Autodesk Fusion 360 part; units mm, degrees
(part 3 of 8)
  spline S623 degree 3 poles (3.0732, -97.2295) (3.0688, -97.132) (3.0596, -97.098) (3.0422, -97.1202) knots 0 0 0 0 1 1 1 1
  spline S624 degree 3 poles (3.0422, -97.1202) (3.0378, -97.1258) (3.0439, -97.1753) (3.0534, -97.2319) knots 0 0 0 0 1 1 1 1
  spline S625 degree 3 poles (10.0535, -88.2722) (10.072, -88.3001) (10.1317, -88.3154) (10.1877, -88.301) knots 0 0 0 0 1 1 1 1
  spline S626 degree 3 poles (10.1877, -88.301) (10.2366, -88.2899) (10.2509, -88.2832) (10.2156, -88.2825) knots 0 0 0 0 1 1 1 1
  spline S627 degree 3 poles (10.2156, -88.2825) (10.1259, -88.2885) (10.0814, -88.2537) (10.1572, -88.2368) knots 0 0 0 0 1 1 1 1
  spline S628 degree 3 poles (10.1572, -88.2368) (10.1913, -88.2276) (10.217, -88.2119) (10.2152, -88.1971) knots 0 0 0 0 1 1 1 1
  spline S629 degree 3 poles (10.2152, -88.1971) (10.2133, -88.1822) (10.2474, -88.173) (10.2898, -88.1703) knots 0 0 0 0 1 1 1 1
  spline S630 degree 3 poles (10.2898, -88.1703) (10.3625, -88.1689) (10.3631, -88.1739) (10.2944, -88.1873) knots 0 0 0 0 1 1 1 1
  spline S631 degree 3 poles (10.2944, -88.1873) (10.1851, -88.2183) (10.2327, -88.2376) (10.4091, -88.2411) knots 0 0 0 0 1 1 1 1
  spline S632 degree 3 poles (10.4091, -88.2411) (10.4895, -88.2413) (10.5632, -88.2272) (10.5635, -88.2096) knots 0 0 0 0 1 1 1 1
  spline S633 degree 3 poles (10.5635, -88.2096) (10.566, -88.1892) (10.5846, -88.1768) (10.61, -88.1787) knots 0 0 0 0 1 1 1 1
  spline S634 degree 3 poles (10.61, -88.1787) (10.6354, -88.1807) (10.6561, -88.1655) (10.6559, -88.1429) knots 0 0 0 0 1 1 1 1
  spline S635 degree 3 poles (10.6559, -88.1429) (10.6593, -88.1099) (10.2729, -88.0945) (10.2138, -88.1243) knots 0 0 0 0 1 1 1 1
  spline S636 degree 3 poles (10.2138, -88.1243) (10.1974, -88.1339) (10.1686, -88.1249) (10.1464, -88.1075) knots 0 0 0 0 1 1 1 1
  spline S637 degree 3 poles (10.1464, -88.1075) (10.0908, -88.0641) (10.0032, -88.2105) (10.0535, -88.2722) knots 0 0 0 0 1 1 1 1
  spline S638 degree 3 poles (10.2393, -88.0458) (10.2449, -88.0502) (10.2845, -88.0453) (10.3257, -88.0327) knots 0 0 0 0 1 1 1 1
  spline S639 degree 3 poles (10.3257, -88.0327) (10.3944, -88.0192) (10.3938, -88.0143) (10.3211, -88.0157) knots 0 0 0 0 1 1 1 1
  spline S640 degree 3 poles (10.3211, -88.0157) (10.2483, -88.0171) (10.2171, -88.0284) (10.2393, -88.0458) knots 0 0 0 0 1 1 1 1
  line L60 (3.056, -97.4578) -> (3.0787, -97.5606)
  line L61 (3.0787, -97.5606) -> (3.0758, -97.4554)
  spline S641 degree 3 poles (3.0758, -97.4554) (3.0713, -97.3981) (3.0652, -97.3486) (3.0596, -97.3442) knots 0 0 0 0 1 1 1 1
  spline S642 degree 3 poles (3.0596, -97.3442) (3.0374, -97.3269) (3.0367, -97.3621) (3.056, -97.4578) knots 0 0 0 0 1 1 1 1
  spline S643 degree 3 poles (10.0643, -88.4016) (10.081, -88.4146) (10.129, -88.4162) (10.1702, -88.4036) knots 0 0 0 0 1 1 1 1
  spline S644 degree 3 poles (10.1702, -88.4036) (10.241, -88.3874) (10.241, -88.3874) (10.1578, -88.3851) knots 0 0 0 0 1 1 1 1
  spline S645 degree 3 poles (10.1578, -88.3851) (10.1099, -88.3834) (10.0619, -88.3818) (10.0542, -88.3802) knots 0 0 0 0 1 1 1 1
  spline S646 degree 3 poles (10.0542, -88.3802) (10.0443, -88.3814) (10.0477, -88.3885) (10.0643, -88.4016) knots 0 0 0 0 1 1 1 1
  spline S647 degree 3 poles (3.0556, -97.6589) (3.0718, -97.7298) (3.0768, -97.7292) (3.0754, -97.6565) knots 0 0 0 0 1 1 1 1
  spline S648 degree 3 poles (3.0754, -97.6565) (3.0755, -97.6162) (3.0706, -97.5766) (3.065, -97.5723) knots 0 0 0 0 1 1 1 1
  spline S649 degree 3 poles (3.065, -97.5723) (3.0428, -97.5549) (3.0393, -97.588) (3.0556, -97.6589) knots 0 0 0 0 1 1 1 1
  spline S650 degree 3 poles (10.9708, -87.4533) (10.9764, -87.4577) (11.016, -87.4528) (11.0572, -87.4402) knots 0 0 0 0 1 1 1 1
  spline S651 degree 3 poles (11.0572, -87.4402) (11.1259, -87.4268) (11.1253, -87.4218) (11.0526, -87.4232) knots 0 0 0 0 1 1 1 1
  spline S652 degree 3 poles (11.0526, -87.4232) (10.9798, -87.4246) (10.9486, -87.436) (10.9708, -87.4533) knots 0 0 0 0 1 1 1 1
  spline S653 degree 3 poles (10.2069, -88.5801) (10.3192, -88.5738) (10.3329, -88.5621) (10.2648, -88.5403) knots 0 0 0 0 1 1 1 1
  spline S654 degree 3 poles (10.2648, -88.5403) (10.2361, -88.5313) (10.1894, -88.5395) (10.1587, -88.5559) knots 0 0 0 0 1 1 1 1
  spline S655 degree 3 poles (10.1587, -88.5559) (10.1165, -88.5811) (10.1249, -88.5876) (10.2069, -88.5801) knots 0 0 0 0 1 1 1 1
  spline S656 degree 3 poles (3.0521, -97.8353) (3.0683, -97.9061) (3.0733, -97.9055) (3.0719, -97.8328) knots 0 0 0 0 1 1 1 1
  spline S657 degree 3 poles (3.0719, -97.8328) (3.072, -97.7926) (3.0671, -97.753) (3.0616, -97.7486) knots 0 0 0 0 1 1 1 1
  spline S658 degree 3 poles (3.0616, -97.7486) (3.0393, -97.7313) (3.0358, -97.7644) (3.0521, -97.8353) knots 0 0 0 0 1 1 1 1
  spline S659 degree 3 poles (11.3124, -87.4516) (11.4105, -87.4521) (11.4974, -87.444) (11.504, -87.4356) knots 0 0 0 0 1 1 1 1
  spline S660 degree 3 poles (11.504, -87.4356) (11.5083, -87.4301) (11.4322, -87.4243) (11.3341, -87.4238) knots 0 0 0 0 1 1 1 1
  spline S661 degree 3 poles (11.3341, -87.4238) (11.236, -87.4233) (11.1491, -87.4315) (11.1426, -87.4398) knots 0 0 0 0 1 1 1 1
  spline S662 degree 3 poles (11.1426, -87.4398) (11.1382, -87.4454) (11.2143, -87.4511) (11.3124, -87.4516) knots 0 0 0 0 1 1 1 1
  spline S663 degree 3 poles (10.5969, -88.2356) (10.6108, -88.2465) (10.6665, -88.2497) (10.7182, -88.2409) knots 0 0 0 0 1 1 1 1
  spline S664 degree 3 poles (10.7182, -88.2409) (10.7699, -88.232) (10.8005, -88.2157) (10.7894, -88.207) knots 0 0 0 0 1 1 1 1
  spline S665 degree 3 poles (10.7894, -88.207) (10.7783, -88.1983) (10.8089, -88.182) (10.8606, -88.1731) knots 0 0 0 0 1 1 1 1
  spline S666 degree 3 poles (10.8606, -88.1731) (10.9123, -88.1642) (10.9652, -88.1653) (10.9819, -88.1783) knots 0 0 0 0 1 1 1 1
  spline S667 degree 3 poles (10.9819, -88.1783) (10.9958, -88.1892) (10.9596, -88.2012) (10.8974, -88.2063) knots 0 0 0 0 1 1 1 1
  spline S668 degree 3 poles (10.8974, -88.2063) (10.7575, -88.2134) (10.8531, -88.2343) (11.0471, -88.2382) knots 0 0 0 0 1 1 1 1
  spline S669 degree 3 poles (11.0471, -88.2382) (11.1275, -88.2383) (11.1891, -88.2283) (11.1873, -88.2134) knots 0 0 0 0 1 1 1 1
  spline S670 degree 3 poles (11.1873, -88.2134) (11.1855, -88.1986) (11.2232, -88.1788) (11.2728, -88.1728) knots 0 0 0 0 1 1 1 1
  spline S671 degree 3 poles (11.2728, -88.1728) (11.3514, -88.1581) (11.3536, -88.1553) (11.3119, -88.1227) knots 0 0 0 0 1 1 1 1
  spline S672 degree 3 poles (11.3119, -88.1227) (11.2841, -88.101) (11.2581, -88.0941) (11.2494, -88.1053) knots 0 0 0 0 1 1 1 1
  spline S673 degree 3 poles (11.2494, -88.1053) (11.2385, -88.1192) (11.1135, -88.1245) (10.9675, -88.1223) knots 0 0 0 0 1 1 1 1
  spline S674 degree 3 poles (10.9675, -88.1223) (10.8236, -88.1173) (10.6964, -88.1254) (10.6856, -88.1393) knots 0 0 0 0 1 1 1 1
  spline S675 degree 3 poles (10.6856, -88.1393) (10.6769, -88.1504) (10.6914, -88.1662) (10.7168, -88.1681) knots 0 0 0 0 1 1 1 1
  spline S676 degree 3 poles (10.7168, -88.1681) (10.7449, -88.1722) (10.7235, -88.1824) (10.6697, -88.194) knots 0 0 0 0 1 1 1 1
  spline S677 degree 3 poles (10.6697, -88.194) (10.613, -88.2035) (10.5802, -88.2226) (10.5969, -88.2356) knots 0 0 0 0 1 1 1 1
  line L62 (3.0493, -98.1196) -> (3.0625, -98.309)
  line L63 (3.0625, -98.309) -> (3.0669, -98.1199)
  spline S678 degree 3 poles (3.0669, -98.1199) (3.0701, -97.9612) (3.0622, -97.8968) (3.0426, -97.9219) knots 0 0 0 0 1 1 1 1
  spline S679 degree 3 poles (3.0426, -97.9219) (3.0383, -97.9274) (3.0415, -98.015) (3.0493, -98.1196) knots 0 0 0 0 1 1 1 1
  spline S680 degree 3 poles (10.3783, -88.5842) (10.4114, -88.5877) (10.4321, -88.6128) (10.4286, -88.6459) knots 0 0 0 0 1 1 1 1
  spline S681 degree 3 poles (10.4286, -88.6459) (10.4251, -88.679) (10.4341, -88.6904) (10.4449, -88.6765) knots 0 0 0 0 1 1 1 1
  spline S682 degree 3 poles (10.4449, -88.6765) (10.458, -88.6598) (10.4686, -88.6234) (10.4699, -88.593) knots 0 0 0 0 1 1 1 1
  spline S683 degree 3 poles (10.4699, -88.593) (10.4749, -88.5522) (10.4588, -88.5441) (10.4, -88.5564) knots 0 0 0 0 1 1 1 1
  spline S684 degree 3 poles (10.4, -88.5564) (10.339, -88.5714) (10.3347, -88.577) (10.3783, -88.5842) knots 0 0 0 0 1 1 1 1
  spline S685 degree 3 poles (7.4661, -92.4377) (7.4741, -92.4618) (7.4886, -92.4776) (7.5035, -92.4758) knots 0 0 0 0 1 1 1 1
  spline S686 degree 3 poles (7.5035, -92.4758) (7.5161, -92.4768) (7.5131, -92.452) (7.4946, -92.4241) knots 0 0 0 0 1 1 1 1
  spline S687 degree 3 poles (7.4946, -92.4241) (7.4625, -92.3677) (7.4412, -92.3779) (7.4661, -92.4377) knots 0 0 0 0 1 1 1 1
  spline S688 degree 3 poles (10.8674, -88.0441) (10.873, -88.0484) (10.9126, -88.0436) (10.9538, -88.031) knots 0 0 0 0 1 1 1 1
  spline S689 degree 3 poles (10.9538, -88.031) (11.0225, -88.0175) (11.0219, -88.0126) (10.9492, -88.0139) knots 0 0 0 0 1 1 1 1
  spline S690 degree 3 poles (10.9492, -88.0139) (10.8765, -88.0153) (10.8452, -88.0267) (10.8674, -88.0441) knots 0 0 0 0 1 1 1 1
  spline S691 degree 3 poles (10.546, -88.5988) (10.5626, -88.6118) (10.5908, -88.6159) (10.6122, -88.6057) knots 0 0 0 0 1 1 1 1
  spline S692 degree 3 poles (10.6122, -88.6057) (10.6335, -88.5956) (10.6246, -88.5841) (10.5958, -88.5751) knots 0 0 0 0 1 1 1 1
  spline S693 degree 3 poles (10.5958, -88.5751) (10.5306, -88.5554) (10.507, -88.5684) (10.546, -88.5988) knots 0 0 0 0 1 1 1 1
  spline S694 degree 3 poles (10.1038, -89.1934) (10.1093, -89.1978) (10.1489, -89.1929) (10.1901, -89.1803) knots 0 0 0 0 1 1 1 1
  spline S695 degree 3 poles (10.1901, -89.1803) (10.2588, -89.1668) (10.2582, -89.1619) (10.1855, -89.1633) knots 0 0 0 0 1 1 1 1
  spline S696 degree 3 poles (10.1855, -89.1633) (10.1128, -89.1647) (10.0815, -89.176) (10.1038, -89.1934) knots 0 0 0 0 1 1 1 1
  spline S697 degree 3 poles (3.0484, -98.5218) (3.0583, -98.6639) (3.0651, -98.6781) (3.0733, -98.5816) knots 0 0 0 0 1 1 1 1
  spline S698 degree 3 poles (3.0733, -98.5816) (3.0813, -98.4625) (3.0607, -98.2941) (3.0439, -98.3213) knots 0 0 0 0 1 1 1 1
  spline S699 degree 3 poles (3.0439, -98.3213) (3.0423, -98.329) (3.0434, -98.4194) (3.0484, -98.5218) knots 0 0 0 0 1 1 1 1
  spline S700 degree 3 poles (11.6264, -87.4508) (11.6787, -87.4468) (11.7255, -87.4386) (11.732, -87.4303) knots 0 0 0 0 1 1 1 1
  spline S701 degree 3 poles (11.732, -87.4303) (11.7385, -87.4219) (11.7005, -87.419) (11.6482, -87.423) knots 0 0 0 0 1 1 1 1
  spline S702 degree 3 poles (11.6482, -87.423) (11.5959, -87.4269) (11.5491, -87.4351) (11.5426, -87.4435) knots 0 0 0 0 1 1 1 1
  spline S703 degree 3 poles (11.5426, -87.4435) (11.5361, -87.4518) (11.5741, -87.4547) (11.6264, -87.4508) knots 0 0 0 0 1 1 1 1
  spline S704 degree 3 poles (11.9405, -87.4499) (12.0386, -87.4504) (12.1255, -87.4423) (12.1321, -87.4339) knots 0 0 0 0 1 1 1 1
  spline S705 degree 3 poles (12.1321, -87.4339) (12.1364, -87.4284) (12.0603, -87.4226) (11.9622, -87.4221) knots 0 0 0 0 1 1 1 1
  spline S706 degree 3 poles (11.9622, -87.4221) (11.8641, -87.4216) (11.7772, -87.4297) (11.7707, -87.4381) knots 0 0 0 0 1 1 1 1
  spline S707 degree 3 poles (11.7707, -87.4381) (11.7663, -87.4436) (11.8424, -87.4494) (11.9405, -87.4499) knots 0 0 0 0 1 1 1 1
  spline S708 degree 3 poles (11.225, -88.2339) (11.2611, -88.2622) (11.4261, -88.2344) (11.4191, -88.1975) knots 0 0 0 0 1 1 1 1
  spline S709 degree 3 poles (11.4191, -88.1975) (11.4164, -88.1551) (11.649, -88.1668) (11.6771, -88.2111) knots 0 0 0 0 1 1 1 1
  spline S710 degree 3 poles (11.6771, -88.2111) (11.69, -88.2346) (11.7342, -88.2468) (11.7732, -88.237) knots 0 0 0 0 1 1 1 1
  spline S711 degree 3 poles (11.7732, -88.237) (11.8101, -88.2299) (11.8308, -88.2148) (11.8197, -88.2061) knots 0 0 0 0 1 1 1 1
  spline S712 degree 3 poles (11.8197, -88.2061) (11.8058, -88.1953) (11.8393, -88.1811) (11.891, -88.1723) knots 0 0 0 0 1 1 1 1
  spline S713 degree 3 poles (11.891, -88.1723) (11.9943, -88.1545) (11.9657, -88.1053) (11.8589, -88.1159) knots 0 0 0 0 1 1 1 1
  spline S714 degree 3 poles (11.8589, -88.1159) (11.8242, -88.1201) (11.7262, -88.1196) (11.6451, -88.1145) knots 0 0 0 0 1 1 1 1
  spline S715 degree 3 poles (11.6451, -88.1145) (11.4428, -88.1041) (11.3586, -88.1145) (11.3656, -88.1513) knots 0 0 0 0 1 1 1 1
  spline S716 degree 3 poles (11.3656, -88.1513) (11.3653, -88.1689) (11.3303, -88.1908) (11.2808, -88.1969) knots 0 0 0 0 1 1 1 1
  spline S717 degree 3 poles (11.2808, -88.1969) (11.234, -88.2052) (11.2083, -88.2209) (11.225, -88.2339) knots 0 0 0 0 1 1 1 1
  spline S718 degree 3 poles (3.0529, -98.8656) (3.0692, -98.9365) (3.0741, -98.9359) (3.0727, -98.8631) knots 0 0 0 0 1 1 1 1
  spline S719 degree 3 poles (3.0727, -98.8631) (3.0728, -98.8229) (3.068, -98.7833) (3.0624, -98.779) knots 0 0 0 0 1 1 1 1
  spline S720 degree 3 poles (3.0624, -98.779) (3.0402, -98.7616) (3.0367, -98.7947) (3.0529, -98.8656) knots 0 0 0 0 1 1 1 1
  spline S721 degree 3 poles (11.446, -88.0484) (11.4516, -88.0528) (11.4912, -88.0479) (11.5324, -88.0353) knots 0 0 0 0 1 1 1 1
  spline S722 degree 3 poles (11.5324, -88.0353) (11.6011, -88.0219) (11.6005, -88.0169) (11.5277, -88.0183) knots 0 0 0 0 1 1 1 1
  spline S723 degree 3 poles (11.5277, -88.0183) (11.455, -88.0197) (11.4238, -88.0311) (11.446, -88.0484) knots 0 0 0 0 1 1 1 1
  spline S724 degree 3 poles (11.2364, -88.5115) (11.2503, -88.5223) (11.2933, -88.5246) (11.3302, -88.5176) knots 0 0 0 0 1 1 1 1
  spline S725 degree 3 poles (11.3302, -88.5176) (11.367, -88.5105) (11.385, -88.4932) (11.3683, -88.4802) knots 0 0 0 0 1 1 1 1
  spline S726 degree 3 poles (11.3683, -88.4802) (11.3544, -88.4694) (11.3114, -88.4671) (11.2746, -88.4741) knots 0 0 0 0 1 1 1 1
  spline S727 degree 3 poles (11.2746, -88.4741) (11.2378, -88.4812) (11.2198, -88.4985) (11.2364, -88.5115) knots 0 0 0 0 1 1 1 1
  spline S728 degree 3 poles (11.4536, -88.2335) (11.4675, -88.2443) (11.5226, -88.2426) (11.5771, -88.2359) knots 0 0 0 0 1 1 1 1
  spline S729 degree 3 poles (11.5771, -88.2359) (11.6777, -88.216) (11.6777, -88.216) (11.5905, -88.2016) knots 0 0 0 0 1 1 1 1
  spline S730 degree 3 poles (11.5905, -88.2016) (11.4977, -88.1828) (11.4147, -88.2031) (11.4536, -88.2335) knots 0 0 0 0 1 1 1 1
  spline S731 degree 3 poles (3.0555, -99.0915) (3.0718, -99.1623) (3.0767, -99.1617) (3.0753, -99.089) knots 0 0 0 0 1 1 1 1
  spline S732 degree 3 poles (3.0753, -99.089) (3.0754, -99.0488) (3.0706, -99.0092) (3.065, -99.0048) knots 0 0 0 0 1 1 1 1
  spline S733 degree 3 poles (3.065, -99.0048) (3.0428, -98.9875) (3.0393, -99.0206) (3.0555, -99.0915) knots 0 0 0 0 1 1 1 1
  spline S734 degree 3 poles (11.0982, -88.7572) (11.1205, -88.7745) (11.1681, -88.7938) (11.2012, -88.7973) knots 0 0 0 0 1 1 1 1
  spline S735 degree 3 poles (11.2012, -88.7973) (11.2773, -88.803) (11.2328, -88.7683) (11.1317, -88.743) knots 0 0 0 0 1 1 1 1
  spline S736 degree 3 poles (11.1317, -88.743) (11.0825, -88.7314) (11.0704, -88.7354) (11.0982, -88.7572) knots 0 0 0 0 1 1 1 1
  spline S737 degree 3 poles (11.6719, -88.0458) (11.6774, -88.0502) (11.717, -88.0453) (11.7582, -88.0327) knots 0 0 0 0 1 1 1 1
  spline S738 degree 3 poles (11.7582, -88.0327) (11.8269, -88.0193) (11.8263, -88.0143) (11.7536, -88.0157) knots 0 0 0 0 1 1 1 1
  spline S739 degree 3 poles (11.7536, -88.0157) (11.6809, -88.0171) (11.6496, -88.0285) (11.6719, -88.0458) knots 0 0 0 0 1 1 1 1
  spline S740 degree 3 poles (12.0628, -87.5455) (12.0684, -87.5498) (12.108, -87.5449) (12.1492, -87.5323) knots 0 0 0 0 1 1 1 1
  spline S741 degree 3 poles (12.1492, -87.5323) (12.2179, -87.5189) (12.2173, -87.5139) (12.1446, -87.5153) knots 0 0 0 0 1 1 1 1
  spline S742 degree 3 poles (12.1446, -87.5153) (12.0719, -87.5167) (12.0406, -87.5281) (12.0628, -87.5455) knots 0 0 0 0 1 1 1 1
  spline S743 degree 3 poles (12.503, -87.4462) (12.697, -87.45) (12.9306, -87.449) (13.0203, -87.443) knots 0 0 0 0 1 1 1 1
  spline S744 degree 3 poles (13.0203, -87.443) (13.1101, -87.437) (13.0263, -87.4297) (12.8323, -87.4259) knots 0 0 0 0 1 1 1 1
  spline S745 degree 3 poles (12.8323, -87.4259) (12.6383, -87.422) (12.4047, -87.4231) (12.3149, -87.4291) knots 0 0 0 0 1 1 1 1
  spline S746 degree 3 poles (12.3149, -87.4291) (12.223, -87.4378) (12.309, -87.4423) (12.503, -87.4462) knots 0 0 0 0 1 1 1 1
  spline S747 degree 3 poles (3.052, -99.2678) (3.0683, -99.3387) (3.0732, -99.3381) (3.0719, -99.2654) knots 0 0 0 0 1 1 1 1
  spline S748 degree 3 poles (3.0719, -99.2654) (3.0719, -99.2252) (3.0671, -99.1855) (3.0615, -99.1812) knots 0 0 0 0 1 1 1 1
  spline S749 degree 3 poles (3.0615, -99.1812) (3.0393, -99.1638) (3.0358, -99.1969) (3.052, -99.2678) knots 0 0 0 0 1 1 1 1
  line L64 (3.0516, -99.4689) -> (3.0743, -99.5717)
  line L65 (3.0743, -99.5717) -> (3.0714, -99.4665)
  spline S750 degree 3 poles (3.0714, -99.4665) (3.067, -99.369) (3.0578, -99.335) (3.0404, -99.3572) knots 0 0 0 0 1 1 1 1
  spline S751 degree 3 poles (3.0404, -99.3572) (3.0361, -99.3628) (3.0421, -99.4123) (3.0516, -99.4689) knots 0 0 0 0 1 1 1 1
  spline S752 degree 3 poles (11.8977, -88.0432) (11.9033, -88.0476) (11.9429, -88.0427) (11.9841, -88.0301) knots 0 0 0 0 1 1 1 1
  spline S753 degree 3 poles (11.9841, -88.0301) (12.0528, -88.0167) (12.0522, -88.0117) (11.9795, -88.0131) knots 0 0 0 0 1 1 1 1
  spline S754 degree 3 poles (11.9795, -88.0131) (11.9068, -88.0145) (11.8755, -88.0259) (11.8977, -88.0432) knots 0 0 0 0 1 1 1 1
  spline S755 degree 3 poles (11.8531, -88.2322) (11.867, -88.2431) (11.9227, -88.2463) (11.9744, -88.2374) knots 0 0 0 0 1 1 1 1
  spline S756 degree 3 poles (11.9744, -88.2374) (12.0261, -88.2286) (12.0567, -88.2122) (12.0456, -88.2035) knots 0 0 0 0 1 1 1 1
  spline S757 degree 3 poles (12.0456, -88.2035) (12.0345, -88.1948) (12.0651, -88.1785) (12.1168, -88.1697) knots 0 0 0 0 1 1 1 1
  spline S758 degree 3 poles (12.1168, -88.1697) (12.2252, -88.1513) (12.1977, -88.112) (12.0715, -88.1074) knots 0 0 0 0 1 1 1 1
  spline S759 degree 3 poles (12.0715, -88.1074) (12.0263, -88.1079) (11.9879, -88.1227) (11.9931, -88.1446) knots 0 0 0 0 1 1 1 1
  spline S760 degree 3 poles (11.9931, -88.1446) (11.9956, -88.1644) (11.9584, -88.1891) (11.9089, -88.1952) knots 0 0 0 0 1 1 1 1
  spline S761 degree 3 poles (11.9089, -88.1952) (11.8621, -88.2034) (11.8364, -88.2192) (11.8531, -88.2322) knots 0 0 0 0 1 1 1 1
  line L66 (3.0542, -99.6948) -> (3.0769, -99.7976)
  line L67 (3.0769, -99.7976) -> (3.074, -99.6924)
  spline S762 degree 3 poles (3.074, -99.6924) (3.0696, -99.5949) (3.0604, -99.5608) (3.043, -99.5831) knots 0 0 0 0 1 1 1 1
  spline S763 degree 3 poles (3.043, -99.5831) (3.0387, -99.5886) (3.0447, -99.6382) (3.0542, -99.6948) knots 0 0 0 0 1 1 1 1
  spline S764 degree 3 poles (12.0741, -88.0467) (12.0797, -88.0511) (12.1193, -88.0462) (12.1605, -88.0336) knots 0 0 0 0 1 1 1 1
  spline S765 degree 3 poles (12.1605, -88.0336) (12.2292, -88.0201) (12.2286, -88.0152) (12.1558, -88.0166) knots 0 0 0 0 1 1 1 1
  spline S766 degree 3 poles (12.1558, -88.0166) (12.0831, -88.018) (12.0519, -88.0293) (12.0741, -88.0467) knots 0 0 0 0 1 1 1 1
  spline S767 degree 3 poles (12.0706, -88.2231) (12.1095, -88.2535) (12.4422, -88.2403) (12.4478, -88.2044) knots 0 0 0 0 1 1 1 1
  spline S768 degree 3 poles (12.4478, -88.2044) (12.4482, -88.1868) (12.4866, -88.172) (12.5296, -88.1743) knots 0 0 0 0 1 1 1 1
  spline S769 degree 3 poles (12.5296, -88.1743) (12.5995, -88.1707) (12.6001, -88.1757) (12.5314, -88.1891) knots 0 0 0 0 1 1 1 1
  spline S770 degree 3 poles (12.5314, -88.1891) (12.4902, -88.2017) (12.4673, -88.2196) (12.484, -88.2326) knots 0 0 0 0 1 1 1 1
  spline S771 degree 3 poles (12.484, -88.2326) (12.5173, -88.2587) (12.6328, -88.237) (12.6285, -88.2023) knots 0 0 0 0 1 1 1 1
  spline S772 degree 3 poles (12.6285, -88.2023) (12.6267, -88.1875) (12.6608, -88.1783) (12.7032, -88.1756) knots 0 0 0 0 1 1 1 1
  spline S773 degree 3 poles (12.7032, -88.1756) (12.7759, -88.1742) (12.7765, -88.1791) (12.7078, -88.1926) knots 0 0 0 0 1 1 1 1
  spline S774 degree 3 poles (12.7078, -88.1926) (12.6666, -88.2052) (12.6436, -88.2231) (12.6603, -88.2361) knots 0 0 0 0 1 1 1 1
  spline S775 degree 3 poles (12.6603, -88.2361) (12.6937, -88.2622) (12.8091, -88.2405) (12.8049, -88.2058) knots 0 0 0 0 1 1 1 1
  spline S776 degree 3 poles (12.8049, -88.2058) (12.8031, -88.191) (12.8371, -88.1817) (12.8795, -88.1791) knots 0 0 0 0 1 1 1 1
  spline S777 degree 3 poles (12.8795, -88.1791) (12.9522, -88.1777) (12.9528, -88.1826) (12.8841, -88.1961) knots 0 0 0 0 1 1 1 1
  spline S778 degree 3 poles (12.8841, -88.1961) (12.8429, -88.2087) (12.82, -88.2266) (12.8339, -88.2374) knots 0 0 0 0 1 1 1 1
  spline S779 degree 3 poles (12.8339, -88.2374) (12.8756, -88.27) (13.0344, -88.2329) (13.0295, -88.1933) knots 0 0 0 0 1 1 1 1
  spline S780 degree 3 poles (13.0295, -88.1933) (13.0271, -88.1735) (13.041, -88.1844) (13.0629, -88.2194) knots 0 0 0 0 1 1 1 1
  spline S781 degree 3 poles (13.0629, -88.2194) (13.0977, -88.2779) (13.0956, -88.2807) (13.0068, -88.274) knots 0 0 0 0 1 1 1 1
  spline S782 degree 3 poles (13.0068, -88.274) (12.956, -88.2702) (12.9043, -88.279) (12.8935, -88.2929) knots 0 0 0 0 1 1 1 1
  spline S783 degree 3 poles (12.8935, -88.2929) (12.8826, -88.3068) (13.0194, -88.3152) (13.1923, -88.3115) knots 0 0 0 0 1 1 1 1
  spline S784 degree 3 poles (13.1923, -88.3115) (13.3681, -88.3101) (13.5095, -88.2952) (13.5077, -88.2804) knots 0 0 0 0 1 1 1 1
  spline S785 degree 3 poles (13.5077, -88.2804) (13.5059, -88.2655) (13.5437, -88.2458) (13.5932, -88.2397) knots 0 0 0 0 1 1 1 1
  spline S786 degree 3 poles (13.5932, -88.2397) (13.6399, -88.2315) (13.6684, -88.2179) (13.6545, -88.207) knots 0 0 0 0 1 1 1 1
  spline S787 degree 3 poles (13.6545, -88.207) (13.6434, -88.1984) (13.6642, -88.1832) (13.701, -88.1762) knots 0 0 0 0 1 1 1 1
  spline S788 degree 3 poles (13.701, -88.1762) (13.7549, -88.1646) (13.7614, -88.1562) (13.7308, -88.1323) knots 0 0 0 0 1 1 1 1
  spline S789 degree 3 poles (13.7308, -88.1323) (13.673, -88.0917) (13.4341, -88.111) (13.4099, -88.1592) knots 0 0 0 0 1 1 1 1
  spline S790 degree 3 poles (13.4099, -88.1592) (13.4024, -88.1802) (13.3705, -88.1866) (13.3461, -88.172) knots 0 0 0 0 1 1 1 1
  spline S791 degree 3 poles (13.3461, -88.172) (13.3239, -88.1546) (13.2834, -88.132) (13.2611, -88.1146) knots 0 0 0 0 1 1 1 1
  spline S792 degree 3 poles (13.2611, -88.1146) (13.2395, -88.1022) (13.2132, -88.1129) (13.202, -88.1445) knots 0 0 0 0 1 1 1 1
  spline S793 degree 3 poles (13.202, -88.1445) (13.1957, -88.1754) (13.1678, -88.1939) (13.1425, -88.192) knots 0 0 0 0 1 1 1 1
  spline S794 degree 3 poles (13.1425, -88.192) (13.1143, -88.1879) (13.1137, -88.183) (13.14, -88.1722) knots 0 0 0 0 1 1 1 1
  spline S795 degree 3 poles (13.14, -88.1722) (13.1664, -88.1614) (13.1772, -88.1475) (13.1633, -88.1367) knots 0 0 0 0 1 1 1 1
  spline S796 degree 3 poles (13.1633, -88.1367) (13.125, -88.1112) (12.9363, -88.0891) (12.9647, -88.1158) knots 0 0 0 0 1 1 1 1
  spline S797 degree 3 poles (12.9647, -88.1158) (12.9786, -88.1267) (12.9341, -88.1321) (12.8623, -88.1208) knots 0 0 0 0 1 1 1 1
  spline S798 degree 3 poles (12.8623, -88.1208) (12.7299, -88.1069) (12.617, -88.1082) (12.4149, -88.1205) knots 0 0 0 0 1 1 1 1
  spline S799 degree 3 poles (12.4149, -88.1205) (12.3499, -88.1234) (12.2794, -88.122) (12.2584, -88.1146) knots 0 0 0 0 1 1 1 1
  spline S800 degree 3 poles (12.2584, -88.1146) (12.2346, -88.1049) (12.216, -88.1173) (12.2184, -88.1371) knots 0 0 0 0 1 1 1 1
  spline S801 degree 3 poles (12.2184, -88.1371) (12.2208, -88.1569) (12.2458, -88.1764) (12.2789, -88.1799) knots 0 0 0 0 1 1 1 1
  spline S802 degree 3 poles (12.2789, -88.1799) (12.3093, -88.1812) (12.2696, -88.1861) (12.1898, -88.1909) knots 0 0 0 0 1 1 1 1
  spline S803 degree 3 poles (12.1898, -88.1909) (12.1128, -88.1978) (12.0567, -88.2122) (12.0706, -88.2231) knots 0 0 0 0 1 1 1 1
  spline S804 degree 3 poles (13.2554, -88.1907) (13.253, -88.1709) (13.2641, -88.1796) (13.2798, -88.2053) knots 0 0 0 0 1 1 1 1
  spline S805 degree 3 poles (13.2798, -88.2053) (13.2983, -88.2332) (13.3432, -88.2503) (13.3822, -88.2405) knots 0 0 0 0 1 1 1 1
  spline S806 degree 3 poles (13.3822, -88.2405) (13.419, -88.2334) (13.4648, -88.2379) (13.4815, -88.2509) knots 0 0 0 0 1 1 1 1
  spline S807 degree 3 poles (13.4815, -88.2509) (13.4981, -88.2639) (13.4272, -88.2802) (13.3248, -88.2852) knots 0 0 0 0 1 1 1 1
  spline S808 degree 3 poles (13.3248, -88.2852) (13.1271, -88.2919) (13.0309, -88.266) (13.1711, -88.2413) knots 0 0 0 0 1 1 1 1
  spline S809 degree 3 poles (13.1711, -88.2413) (13.2207, -88.2352) (13.2578, -88.2105) (13.2554, -88.1907) knots 0 0 0 0 1 1 1 1
  spline S810 degree 3 poles (13.5571, -88.1712) (13.6298, -88.1699) (13.6304, -88.1748) (13.5617, -88.1883) knots 0 0 0 0 1 1 1 1
  spline S811 degree 3 poles (13.5617, -88.1883) (13.5206, -88.2009) (13.4809, -88.2057) (13.4754, -88.2014) knots 0 0 0 0 1 1 1 1
  spline S812 degree 3 poles (13.4754, -88.2014) (13.4531, -88.184) (13.4844, -88.1726) (13.5571, -88.1712) knots 0 0 0 0 1 1 1 1
  spline S813 degree 3 poles (3.0538, -99.8959) (3.07, -99.9668) (3.075, -99.9662) (3.0736, -99.8935) knots 0 0 0 0 1 1 1 1
  spline S814 degree 3 poles (3.0736, -99.8935) (3.0722, -99.8208) (3.0608, -99.7895) (3.0434, -99.8117) knots 0 0 0 0 1 1 1 1
  spline S815 degree 3 poles (3.0434, -99.8117) (3.0391, -99.8173) (3.044, -99.8569) (3.0538, -99.8959) knots 0 0 0 0 1 1 1 1
  spline S816 degree 3 poles (12.3, -88.0441) (12.3055, -88.0485) (12.3451, -88.0436) (12.3863, -88.031) knots 0 0 0 0 1 1 1 1
  spline S817 degree 3 poles (12.3863, -88.031) (12.455, -88.0175) (12.4544, -88.0126) (12.3817, -88.014) knots 0 0 0 0 1 1 1 1
  spline S818 degree 3 poles (12.3817, -88.014) (12.309, -88.0154) (12.2777, -88.0267) (12.3, -88.0441) knots 0 0 0 0 1 1 1 1
  spline S819 degree 3 poles (12.1952, -88.4189) (12.2929, -88.4371) (12.4254, -88.4107) (12.3893, -88.3825) knots 0 0 0 0 1 1 1 1
  spline S820 degree 3 poles (12.3893, -88.3825) (12.3754, -88.3716) (12.3076, -88.3724) (12.2383, -88.3809) knots 0 0 0 0 1 1 1 1
  spline S821 degree 3 poles (12.2383, -88.3809) (12.1278, -88.402) (12.1207, -88.4054) (12.1952, -88.4189) knots 0 0 0 0 1 1 1 1
  spline S822 degree 3 poles (12.9548, -87.544) (12.9892, -87.5574) (13.0161, -87.5516) (13.0143, -87.5367) knots 0 0 0 0 1 1 1 1
  spline S823 degree 3 poles (13.0143, -87.5367) (13.0124, -87.5219) (12.9837, -87.5128) (12.949, -87.5171) knots 0 0 0 0 1 1 1 1
  spline S824 degree 3 poles (12.949, -87.5171) (12.9023, -87.5253) (12.9029, -87.5303) (12.9548, -87.544) knots 0 0 0 0 1 1 1 1
  spline S825 degree 3 poles (8.8233, -92.9295) (8.8622, -92.9599) (8.8805, -92.9652) (8.8675, -92.9417) knots 0 0 0 0 1 1 1 1
  spline S826 degree 3 poles (8.8675, -92.9417) (8.8552, -92.9231) (8.8219, -92.897) (8.7981, -92.8874) knots 0 0 0 0 1 1 1 1
  spline S827 degree 3 poles (8.7981, -92.8874) (8.7749, -92.8827) (8.7844, -92.8991) (8.8233, -92.9295) knots 0 0 0 0 1 1 1 1
  spline S828 degree 3 poles (11.7611, -89.1407) (11.7916, -89.1646) (11.8677, -89.1704) (11.9281, -89.1504) knots 0 0 0 0 1 1 1 1
  line L68 (11.9281, -89.1504) -> (12.0396, -89.1166)
  line L69 (12.0396, -89.1166) -> (11.9273, -89.1228)
  spline S829 degree 3 poles (11.9273, -89.1228) (11.8651, -89.128) (11.789, -89.1222) (11.7602, -89.1132) knots 0 0 0 0 1 1 1 1
  spline S830 degree 3 poles (11.7602, -89.1132) (11.7209, -89.1004) (11.7221, -89.1103) (11.7611, -89.1407) knots 0 0 0 0 1 1 1 1
  spline S831 degree 3 poles (3.1459, -100.2365) (3.1621, -100.3073) (3.167, -100.3067) (3.1657, -100.234) knots 0 0 0 0 1 1 1 1
  spline S832 degree 3 poles (3.1657, -100.234) (3.1657, -100.1938) (3.1609, -100.1542) (3.1553, -100.1498) knots 0 0 0 0 1 1 1 1
  spline S833 degree 3 poles (3.1553, -100.1498) (3.1331, -100.1325) (3.1296, -100.1656) (3.1459, -100.2365) knots 0 0 0 0 1 1 1 1
  spline S834 degree 3 poles (8.3425, -93.6596) (8.3498, -93.6788) (8.3724, -93.6785) (8.3898, -93.6563) knots 0 0 0 0 1 1 1 1
  spline S835 degree 3 poles (8.3898, -93.6563) (8.4094, -93.6313) (8.4107, -93.6009) (8.3968, -93.5901) knots 0 0 0 0 1 1 1 1
  spline S836 degree 3 poles (8.3968, -93.5901) (8.3801, -93.5771) (8.3603, -93.5795) (8.3494, -93.5934) knots 0 0 0 0 1 1 1 1
  spline S837 degree 3 poles (8.3494, -93.5934) (8.3364, -93.6101) (8.3323, -93.6382) (8.3425, -93.6596) knots 0 0 0 0 1 1 1 1
  spline S838 degree 3 poles (13.2849, -87.4482) (13.3372, -87.4443) (13.3839, -87.436) (13.3904, -87.4277) knots 0 0 0 0 1 1 1 1
  spline S839 degree 3 poles (13.3904, -87.4277) (13.3969, -87.4193) (13.3589, -87.4165) (13.3066, -87.4204) knots 0 0 0 0 1 1 1 1
  spline S840 degree 3 poles (13.3066, -87.4204) (13.2543, -87.4243) (13.2076, -87.4325) (13.201, -87.4409) knots 0 0 0 0 1 1 1 1
  spline S841 degree 3 poles (13.201, -87.4409) (13.1945, -87.4492) (13.2326, -87.4521) (13.2849, -87.4482) knots 0 0 0 0 1 1 1 1
  spline S842 degree 3 poles (12.351, -88.6436) (12.3714, -88.6461) (12.3961, -88.643) (12.4026, -88.6347) knots 0 0 0 0 1 1 1 1
  spline S843 degree 3 poles (12.4026, -88.6347) (12.407, -88.6291) (12.3974, -88.6127) (12.3835, -88.6019) knots 0 0 0 0 1 1 1 1
  spline S844 degree 3 poles (12.3835, -88.6019) (12.3669, -88.5888) (12.3449, -88.594) (12.3318, -88.6107) knots 0 0 0 0 1 1 1 1
  spline S845 degree 3 poles (12.3318, -88.6107) (12.321, -88.6246) (12.3278, -88.6389) (12.351, -88.6436) knots 0 0 0 0 1 1 1 1
  spline S846 degree 3 poles (8.9986, -93.0261) (9.0291, -93.05) (9.044, -93.0482) (9.0283, -93.0225) knots 0 0 0 0 1 1 1 1
  spline S847 degree 3 poles (9.0283, -93.0225) (9.0153, -92.9989) (8.9881, -92.9822) (8.9733, -92.984) knots 0 0 0 0 1 1 1 1
  spline S848 degree 3 poles (8.9733, -92.984) (8.9556, -92.9836) (8.9658, -93.005) (8.9986, -93.0261) knots 0 0 0 0 1 1 1 1
  spline S849 degree 3 poles (12.8786, -88.0485) (12.8841, -88.0528) (12.9237, -88.048) (12.9649, -88.0354) knots 0 0 0 0 1 1 1 1
  spline S850 degree 3 poles (12.9649, -88.0354) (13.0336, -88.0219) (13.033, -88.0169) (12.9603, -88.0183) knots 0 0 0 0 1 1 1 1
  spline S851 degree 3 poles (12.9603, -88.0183) (12.8876, -88.0197) (12.8563, -88.0311) (12.8786, -88.0485) knots 0 0 0 0 1 1 1 1
  spline S852 degree 3 poles (13.4337, -87.4525) (13.4393, -87.4569) (13.4789, -87.452) (13.52, -87.4394) knots 0 0 0 0 1 1 1 1
  spline S853 degree 3 poles (13.52, -87.4394) (13.5888, -87.426) (13.5882, -87.421) (13.5154, -87.4224) knots 0 0 0 0 1 1 1 1
  spline S854 degree 3 poles (13.5154, -87.4224) (13.4427, -87.4238) (13.4115, -87.4352) (13.4337, -87.4525) knots 0 0 0 0 1 1 1 1
  spline S855 degree 3 poles (13.6871, -87.4491) (13.7394, -87.4452) (13.7861, -87.4369) (13.7927, -87.4286) knots 0 0 0 0 1 1 1 1
  spline S856 degree 3 poles (13.7927, -87.4286) (13.7992, -87.4202) (13.7611, -87.4174) (13.7088, -87.4213) knots 0 0 0 0 1 1 1 1
  spline S857 degree 3 poles (13.7088, -87.4213) (13.6565, -87.4252) (13.6098, -87.4334) (13.6033, -87.4418) knots 0 0 0 0 1 1 1 1
  spline S858 degree 3 poles (13.6033, -87.4418) (13.5968, -87.4501) (13.6348, -87.453) (13.6871, -87.4491) knots 0 0 0 0 1 1 1 1
  spline S859 degree 3 poles (9.2405, -93.1748) (9.2683, -93.1966) (9.3236, -93.2174) (9.3567, -93.2209) knots 0 0 0 0 1 1 1 1
  spline S860 degree 3 poles (9.3567, -93.2209) (9.4047, -93.2225) (9.3957, -93.2111) (9.3237, -93.1772) knots 0 0 0 0 1 1 1 1
  spline S861 degree 3 poles (9.3237, -93.1772) (9.2035, -93.1191) (9.1682, -93.1184) (9.2405, -93.1748) knots 0 0 0 0 1 1 1 1
  spline S862 degree 3 poles (11.5894, -90.2601) (11.6283, -90.2905) (11.678, -90.3472) (11.6993, -90.3773) knots 0 0 0 0 1 1 1 1
  spline S863 degree 3 poles (11.6993, -90.3773) (11.7357, -90.4281) (11.7357, -90.4281) (11.7123, -90.3606) knots 0 0 0 0 1 1 1 1
  spline S864 degree 3 poles (11.7123, -90.3606) (11.6975, -90.3222) (11.6485, -90.2704) (11.6024, -90.2434) knots 0 0 0 0 1 1 1 1
  line L70 (11.6024, -90.2434) -> (11.5187, -90.1959)
  line L71 (11.5187, -90.1959) -> (11.5894, -90.2601)
  spline S865 degree 3 poles (14.2552, -87.4497) (14.675, -87.4509) (14.978, -87.4414) (14.8886, -87.4297) knots 0 0 0 0 1 1 1 1
  spline S866 degree 3 poles (14.8886, -87.4297) (14.802, -87.4202) (13.8422, -87.4225) (13.8335, -87.4336) knots 0 0 0 0 1 1 1 1
  spline S867 degree 3 poles (13.8335, -87.4336) (13.827, -87.4419) (14.0188, -87.4486) (14.2552, -87.4497) knots 0 0 0 0 1 1 1 1
  spline S868 degree 3 poles (7.0992, -96.225) (7.0802, -96.2951) (7.083, -96.2973) (7.1308, -96.2362) knots 0 0 0 0 1 1 1 1
  spline S869 degree 3 poles (7.1308, -96.2362) (7.1596, -96.205) (7.1674, -96.1663) (7.1535, -96.1555) knots 0 0 0 0 1 1 1 1
  spline S870 degree 3 poles (7.1535, -96.1555) (7.1369, -96.1424) (7.1236, -96.1365) (7.1242, -96.1415) knots 0 0 0 0 1 1 1 1
  spline S871 degree 3 poles (7.1242, -96.1415) (7.1198, -96.147) (7.1092, -96.1835) (7.0992, -96.225) knots 0 0 0 0 1 1 1 1
  spline S872 degree 3 poles (12.2141, -89.6782) (12.2454, -89.6668) (12.2853, -89.6443) (12.2962, -89.6304) knots 0 0 0 0 1 1 1 1
  spline S873 degree 3 poles (12.2962, -89.6304) (12.3092, -89.6138) (12.2888, -89.6112) (12.2575, -89.6226) knots 0 0 0 0 1 1 1 1
  spline S874 degree 3 poles (12.2575, -89.6226) (12.2263, -89.634) (12.1885, -89.6537) (12.1754, -89.6704) knots 0 0 0 0 1 1 1 1
  spline S875 degree 3 poles (12.1754, -89.6704) (12.1646, -89.6843) (12.1828, -89.6896) (12.2141, -89.6782) knots 0 0 0 0 1 1 1 1
  spline S876 degree 3 poles (9.4501, -93.2446) (9.464, -93.2555) (9.5215, -93.2735) (9.5778, -93.2817) knots 0 0 0 0 1 1 1 1
  spline S877 degree 3 poles (9.5778, -93.2817) (9.6341, -93.2899) (9.6638, -93.2862) (9.6499, -93.2754) knots 0 0 0 0 1 1 1 1
  spline S878 degree 3 poles (9.6499, -93.2754) (9.6333, -93.2623) (9.5785, -93.2464) (9.5222, -93.2383) knots 0 0 0 0 1 1 1 1
  spline S879 degree 3 poles (9.5222, -93.2383) (9.4659, -93.2301) (9.4334, -93.2316) (9.4501, -93.2446) knots 0 0 0 0 1 1 1 1
  spline S880 degree 3 poles (13.5067, -88.0468) (13.5122, -88.0511) (13.5518, -88.0462) (13.593, -88.0336) knots 0 0 0 0 1 1 1 1
  spline S881 degree 3 poles (13.593, -88.0336) (13.6617, -88.0202) (13.6611, -88.0152) (13.5884, -88.0166) knots 0 0 0 0 1 1 1 1
  spline S882 degree 3 poles (13.5884, -88.0166) (13.5157, -88.018) (13.4844, -88.0294) (13.5067, -88.0468) knots 0 0 0 0 1 1 1 1
  spline S883 degree 3 poles (12.4514, -89.9532) (12.5572, -90.1388) (12.5907, -90.2276) (12.56, -90.244) knots 0 0 0 0 1 1 1 1
  spline S884 degree 3 poles (12.56, -90.244) (12.5343, -90.2597) (12.5268, -90.2807) (12.5407, -90.2916) knots 0 0 0 0 1 1 1 1
  spline S885 degree 3 poles (12.5407, -90.2916) (12.5574, -90.3046) (12.5772, -90.3022) (12.5903, -90.2855) knots 0 0 0 0 1 1 1 1
  spline S886 degree 3 poles (12.5903, -90.2855) (12.6011, -90.2716) (12.6221, -90.2791) (12.6351, -90.3026) knots 0 0 0 0 1 1 1 1
  spline S887 degree 3 poles (12.6351, -90.3026) (12.6502, -90.3234) (12.7071, -90.3365) (12.7637, -90.327) knots 0 0 0 0 1 1 1 1
  spline S888 degree 3 poles (12.7637, -90.327) (12.8643, -90.3071) (12.8643, -90.3071) (12.7777, -90.2977) knots 0 0 0 0 1 1 1 1
  spline S889 degree 3 poles (12.7777, -90.2977) (12.7038, -90.2891) (12.6692, -90.2532) (12.5462, -90.0496) knots 0 0 0 0 1 1 1 1
  spline S890 degree 3 poles (12.5462, -90.0496) (12.3076, -89.6617) (12.31, -89.6815) (12.5096, -89.6495) knots 0 0 0 0 1 1 1 1
  line L72 (12.5096, -89.6495) -> (12.6845, -89.6205)
  line L73 (12.6845, -89.6205) -> (12.505, -89.6324)
  spline S891 degree 3 poles (12.505, -89.6324) (12.4082, -89.6418) (12.3197, -89.6577) (12.311, -89.6688) knots 0 0 0 0 1 1 1 1
  spline S892 degree 3 poles (12.311, -89.6688) (12.3023, -89.68) (12.3654, -89.8054) (12.4514, -89.9532) knots 0 0 0 0 1 1 1 1
  spline S893 degree 3 poles (11.7658, -90.5099) (11.8185, -90.5914) (11.8396, -90.5988) (11.81, -90.522) knots 0 0 0 0 1 1 1 1
  spline S894 degree 3 poles (11.81, -90.522) (11.7953, -90.4836) (11.7712, -90.4514) (11.7591, -90.4554) knots 0 0 0 0 1 1 1 1
  spline S895 degree 3 poles (11.7591, -90.4554) (11.7464, -90.4544) (11.7495, -90.4792) (11.7658, -90.5099) knots 0 0 0 0 1 1 1 1
  spline S896 degree 3 poles (13.7325, -88.0442) (13.7381, -88.0485) (13.7777, -88.0436) (13.8189, -88.031) knots 0 0 0 0 1 1 1 1
  spline S897 degree 3 poles (13.8189, -88.031) (13.8876, -88.0176) (13.887, -88.0126) (13.8143, -88.014) knots 0 0 0 0 1 1 1 1
  spline S898 degree 3 poles (13.8143, -88.014) (13.7416, -88.0154) (13.7103, -88.0268) (13.7325, -88.0442) knots 0 0 0 0 1 1 1 1
  spline S899 degree 3 poles (3.8616, -100.7643) (3.8414, -100.8246) (3.8469, -100.829) (3.8918, -100.8058) knots 0 0 0 0 1 1 1 1
  spline S900 degree 3 poles (3.8918, -100.8058) (3.9219, -100.7846) (3.9331, -100.753) (3.9146, -100.7251) knots 0 0 0 0 1 1 1 1
  spline S901 degree 3 poles (3.9146, -100.7251) (3.8989, -100.6994) (3.8844, -100.6836) (3.885, -100.6886) knots 0 0 0 0 1 1 1 1
  spline S902 degree 3 poles (3.885, -100.6886) (3.8828, -100.6913) (3.8722, -100.7278) (3.8616, -100.7643) knots 0 0 0 0 1 1 1 1
  spline S903 degree 3 poles (13.6934, -88.2374) (13.7129, -88.2527) (13.7076, -88.2709) (13.6813, -88.2817) knots 0 0 0 0 1 1 1 1
  spline S904 degree 3 poles (13.6813, -88.2817) (13.6549, -88.2924) (13.6484, -88.3008) (13.6682, -88.2983) knots 0 0 0 0 1 1 1 1
  spline S905 degree 3 poles (13.6682, -88.2983) (13.6859, -88.2987) (13.7122, -88.2879) (13.7231, -88.274) knots 0 0 0 0 1 1 1 1
  spline S906 degree 3 poles (13.7231, -88.274) (13.7317, -88.2629) (13.7674, -88.246) (13.8014, -88.2368) knots 0 0 0 0 1 1 1 1
  spline S907 degree 3 poles (13.8014, -88.2368) (13.8773, -88.2199) (13.9362, -88.1674) (13.9208, -88.1241) knots 0 0 0 0 1 1 1 1
  spline S908 degree 3 poles (13.9208, -88.1241) (13.9134, -88.1049) (13.8732, -88.1048) (13.8326, -88.1223) knots 0 0 0 0 1 1 1 1
  spline S909 degree 3 poles (13.8326, -88.1223) (13.792, -88.1399) (13.7669, -88.1606) (13.778, -88.1693) knots 0 0 0 0 1 1 1 1
  spline S910 degree 3 poles (13.778, -88.1693) (13.7864, -88.1758) (13.7656, -88.1909) (13.7288, -88.1979) knots 0 0 0 0 1 1 1 1
  spline S911 degree 3 poles (13.7288, -88.1979) (13.6799, -88.209) (13.6712, -88.2201) (13.6934, -88.2374) knots 0 0 0 0 1 1 1 1
  spline S912 degree 3 poles (11.8811, -90.7118) (11.9098, -90.7611) (11.9422, -90.7999) (11.9548, -90.8008) knots 0 0 0 0 1 1 1 1
  spline S913 degree 3 poles (11.9548, -90.8008) (11.9669, -90.7968) (11.9543, -90.7556) (11.9257, -90.7064) knots 0 0 0 0 1 1 1 1
  spline S914 degree 3 poles (11.9257, -90.7064) (11.897, -90.6571) (11.8646, -90.6184) (11.8547, -90.6196) knots 0 0 0 0 1 1 1 1
  spline S915 degree 3 poles (11.8547, -90.6196) (11.8448, -90.6208) (11.8574, -90.662) (11.8811, -90.7118) knots 0 0 0 0 1 1 1 1
  spline S916 degree 3 poles (9.7822, -93.3295) (9.7934, -93.3382) (9.9202, -93.3477) (10.0635, -93.3477) knots 0 0 0 0 1 1 1 1
  spline S917 degree 3 poles (10.0635, -93.3477) (10.237, -93.3491) (10.3348, -93.3672) (10.3622, -93.4066) knots 0 0 0 0 1 1 1 1
  spline S918 degree 3 poles (10.3622, -93.4066) (10.3903, -93.4509) (10.3952, -93.4503) (10.3792, -93.402) knots 0 0 0 0 1 1 1 1
  spline S919 degree 3 poles (10.3792, -93.402) (10.3682, -93.3531) (10.4082, -93.3306) (10.623, -93.279) knots 0 0 0 0 1 1 1 1
  spline S920 degree 3 poles (10.623, -93.279) (10.767, -93.2438) (10.8927, -93.2032) (10.8992, -93.1949) knots 0 0 0 0 1 1 1 1
  spline S921 degree 3 poles (10.8992, -93.1949) (10.9079, -93.1837) (10.7875, -93.2061) (10.6314, -93.2453) knots 0 0 0 0 1 1 1 1
  spline S922 degree 3 poles (10.6314, -93.2453) (10.4754, -93.2846) (10.2179, -93.3162) (10.057, -93.3159) knots 0 0 0 0 1 1 1 1
  spline S923 degree 3 poles (10.057, -93.3159) (9.8961, -93.3155) (9.7739, -93.323) (9.7822, -93.3295) knots 0 0 0 0 1 1 1 1
  spline S924 degree 3 poles (13.9165, -88.2327) (13.9304, -88.2435) (13.9734, -88.2458) (14.0103, -88.2388) knots 0 0 0 0 1 1 1 1
  spline S925 degree 3 poles (14.0103, -88.2388) (14.0471, -88.2317) (14.0679, -88.2166) (14.0567, -88.2079) knots 0 0 0 0 1 1 1 1
  spline S926 degree 3 poles (14.0567, -88.2079) (14.0456, -88.1992) (14.0642, -88.1869) (14.0983, -88.1777) knots 0 0 0 0 1 1 1 1
  spline S927 degree 3 poles (14.0983, -88.1777) (14.1351, -88.1707) (14.1574, -88.1478) (14.15, -88.1286) knots 0 0 0 0 1 1 1 1
  spline S928 degree 3 poles (14.15, -88.1286) (14.1427, -88.1094) (14.0969, -88.105) (14.048, -88.116) knots 0 0 0 0 1 1 1 1
  spline S929 degree 3 poles (14.048, -88.116) (13.9424, -88.1365) (13.9151, -88.16) (13.9841, -88.1691) knots 0 0 0 0 1 1 1 1
  spline S930 degree 3 poles (13.9841, -88.1691) (14.02, -88.1747) (14.0135, -88.1831) (13.9618, -88.1919) knots 0 0 0 0 1 1 1 1
  spline S931 degree 3 poles (13.9618, -88.1919) (13.9228, -88.2017) (13.8998, -88.2196) (13.9165, -88.2327) knots 0 0 0 0 1 1 1 1
  spline S932 degree 3 poles (13.7594, -88.4681) (13.765, -88.4724) (13.8046, -88.4676) (13.8458, -88.455) knots 0 0 0 0 1 1 1 1
  spline S933 degree 3 poles (13.8458, -88.455) (13.9145, -88.4415) (13.9139, -88.4366) (13.8412, -88.438) knots 0 0 0 0 1 1 1 1
  spline S934 degree 3 poles (13.8412, -88.438) (13.7685, -88.4393) (13.7372, -88.4507) (13.7594, -88.4681) knots 0 0 0 0 1 1 1 1
  spline S935 degree 3 poles (14.1348, -88.045) (14.1403, -88.0494) (14.1799, -88.0445) (14.2211, -88.0319) knots 0 0 0 0 1 1 1 1
  spline S936 degree 3 poles (14.2211, -88.0319) (14.2898, -88.0185) (14.2892, -88.0135) (14.2165, -88.0149) knots 0 0 0 0 1 1 1 1
  spline S937 degree 3 poles (14.2165, -88.0149) (14.1438, -88.0163) (14.1125, -88.0277) (14.1348, -88.045) knots 0 0 0 0 1 1 1 1
  spline S938 degree 3 poles (10.0203, -93.4259) (10.0258, -93.4303) (10.0654, -93.4254) (10.1066, -93.4128) knots 0 0 0 0 1 1 1 1
  spline S939 degree 3 poles (10.1066, -93.4128) (10.1753, -93.3994) (10.1747, -93.3944) (10.102, -93.3958) knots 0 0 0 0 1 1 1 1
  spline S940 degree 3 poles (10.102, -93.3958) (10.0293, -93.3972) (9.998, -93.4086) (10.0203, -93.4259) knots 0 0 0 0 1 1 1 1
  spline S941 degree 3 poles (14.0818, -88.2275) (14.129, -88.2644) (14.7303, -88.2283) (14.7353, -88.1874) knots 0 0 0 0 1 1 1 1
  spline S942 degree 3 poles (14.7353, -88.1874) (14.7378, -88.167) (14.7477, -88.1658) (14.7557, -88.19) knots 0 0 0 0 1 1 1 1
  spline S943 degree 3 poles (14.7557, -88.19) (14.7733, -88.2305) (15.5643, -88.4501) (15.5594, -88.4105) knots 0 0 0 0 1 1 1 1
  spline S944 degree 3 poles (15.5594, -88.4105) (15.5604, -88.3978) (15.5028, -88.3797) (15.4333, -88.3656) knots 0 0 0 0 1 1 1 1
  spline S945 degree 3 poles (15.4333, -88.3656) (15.3665, -88.3537) (15.291, -88.3127) (15.2642, -88.2783) knots 0 0 0 0 1 1 1 1
  spline S946 degree 3 poles (15.2642, -88.2783) (15.2306, -88.2297) (15.2229, -88.2281) (15.2354, -88.2693) knots 0 0 0 0 1 1 1 1
  spline S947 degree 3 poles (15.2354, -88.2693) (15.2487, -88.3154) (15.2366, -88.3194) (15.1763, -88.2992) knots 0 0 0 0 1 1 1 1
  spline S948 degree 3 poles (15.1763, -88.2992) (15.1392, -88.2836) (15.0981, -88.256) (15.0907, -88.2368) knots 0 0 0 0 1 1 1 1
  spline S949 degree 3 poles (15.0907, -88.2368) (15.0855, -88.2148) (15.0317, -88.1862) (14.9776, -88.1753) knots 0 0 0 0 1 1 1 1
  spline S950 degree 3 poles (14.9776, -88.1753) (14.8919, -88.1531) (14.8753, -88.1401) (14.8773, -88.0745) knots 0 0 0 0 1 1 1 1
  spline S951 degree 3 poles (14.8773, -88.0745) (14.8793, -88.0089) (14.8731, -87.9996) (14.8121, -88.0146) knots 0 0 0 0 1 1 1 1
  spline S952 degree 3 poles (14.8121, -88.0146) (14.7533, -88.0269) (14.7539, -88.0318) (14.8037, -88.0483) knots 0 0 0 0 1 1 1 1
  spline S953 degree 3 poles (14.8037, -88.0483) (14.843, -88.0611) (14.8503, -88.0803) (14.8243, -88.1137) knots 0 0 0 0 1 1 1 1
  spline S954 degree 3 poles (14.8243, -88.1137) (14.8026, -88.1415) (14.78, -88.1417) (14.7686, -88.1105) knots 0 0 0 0 1 1 1 1
  spline S955 degree 3 poles (14.7686, -88.1105) (14.7606, -88.0863) (14.7523, -88.0798) (14.7525, -88.1024) knots 0 0 0 0 1 1 1 1
  spline S956 degree 3 poles (14.7525, -88.1024) (14.7549, -88.1222) (14.6262, -88.138) (14.4675, -88.1349) knots 0 0 0 0 1 1 1 1
  spline S957 degree 3 poles (14.4675, -88.1349) (14.3066, -88.1345) (14.1794, -88.1426) (14.1812, -88.1574) knots 0 0 0 0 1 1 1 1
  spline S958 degree 3 poles (14.1812, -88.1574) (14.1809, -88.1751) (14.1579, -88.193) (14.1239, -88.2022) knots 0 0 0 0 1 1 1 1
  spline S959 degree 3 poles (14.1239, -88.2022) (14.092, -88.2086) (14.0734, -88.221) (14.0818, -88.2275) knots 0 0 0 0 1 1 1 1
  spline S960 degree 3 poles (14.7038, -88.1762) (14.7177, -88.1871) (14.7211, -88.1942) (14.7112, -88.1954) knots 0 0 0 0 1 1 1 1
  spline S961 degree 3 poles (14.7112, -88.1954) (14.7013, -88.1966) (14.5828, -88.1936) (14.4472, -88.1952) knots 0 0 0 0 1 1 1 1
  line L74 (14.4472, -88.1952) -> (14.2009, -88.1952)
  line L75 (14.2009, -88.1952) -> (14.4399, -88.176)
  spline S962 degree 3 poles (14.4399, -88.176) (14.5692, -88.1651) (14.6899, -88.1654) (14.7038, -88.1762) knots 0 0 0 0 1 1 1 1
  spline S963 degree 3 poles (15.0632, -88.2377) (15.0771, -88.2485) (15.0474, -88.2522) (14.9911, -88.244) knots 0 0 0 0 1 1 1 1
  spline S964 degree 3 poles (14.9911, -88.244) (14.9348, -88.2358) (14.8773, -88.2178) (14.8634, -88.2069) knots 0 0 0 0 1 1 1 1
  spline S965 degree 3 poles (14.8634, -88.2069) (14.8467, -88.1939) (14.8792, -88.1924) (14.9355, -88.2006) knots 0 0 0 0 1 1 1 1
  spline S966 degree 3 poles (14.9355, -88.2006) (14.9918, -88.2087) (15.0465, -88.2246) (15.0632, -88.2377) knots 0 0 0 0 1 1 1 1
  spline S967 degree 3 poles (12.1975, -91.0575) (12.2109, -91.1262) (12.2211, -91.1476) (12.2234, -91.1046) knots 0 0 0 0 1 1 1 1
  spline S968 degree 3 poles (12.2234, -91.1046) (12.2248, -91.0341) (12.2406, -91.0196) (12.3737, -90.9982) knots 0 0 0 0 1 1 1 1
  line L76 (12.3737, -90.9982) -> (12.5238, -90.9722)
  line L77 (12.5238, -90.9722) -> (12.3718, -90.9833)
  spline S969 degree 3 poles (12.3718, -90.9833) (12.292, -90.9881) (12.2175, -90.9746) (12.2073, -90.9533) knots 0 0 0 0 1 1 1 1
  spline S970 degree 3 poles (12.2073, -90.9533) (12.1799, -90.8737) (12.1739, -90.9272) (12.1975, -91.0575) knots 0 0 0 0 1 1 1 1
  spline S971 degree 3 poles (3.924, -101.6413) (3.9546, -101.6652) (3.9695, -101.6634) (3.9537, -101.6377) knots 0 0 0 0 1 1 1 1
  spline S972 degree 3 poles (3.9537, -101.6377) (3.9408, -101.6141) (3.9136, -101.5974) (3.8988, -101.5992) knots 0 0 0 0 1 1 1 1
  spline S973 degree 3 poles (3.8988, -101.5992) (3.8811, -101.5988) (3.8913, -101.6202) (3.924, -101.6413) knots 0 0 0 0 1 1 1 1
  spline S974 degree 3 poles (12.726, -90.593) (12.7704, -90.8113) (12.7895, -90.8441) (12.7741, -90.6977) knots 0 0 0 0 1 1 1 1
  spline S975 degree 3 poles (12.7741, -90.6977) (12.7653, -90.6058) (12.7491, -90.5349) (12.7342, -90.5367) knots 0 0 0 0 1 1 1 1
  spline S976 degree 3 poles (12.7342, -90.5367) (12.7243, -90.5379) (12.7196, -90.5611) (12.726, -90.593) knots 0 0 0 0 1 1 1 1
  spline S977 degree 3 poles (13.57, -89.4841) (13.5839, -89.495) (13.6186, -89.4907) (13.6465, -89.4722) knots 0 0 0 0 1 1 1 1
  spline S978 degree 3 poles (13.6465, -89.4722) (13.6908, -89.4441) (13.6902, -89.4392) (13.6302, -89.4415) knots 0 0 0 0 1 1 1 1
  spline S979 degree 3 poles (13.6302, -89.4415) (13.5525, -89.4435) (13.5339, -89.4559) (13.57, -89.4841) knots 0 0 0 0 1 1 1 1
  spline S980 degree 3 poles (9.9134, -94.193) (9.919, -94.1974) (9.9586, -94.1925) (9.9998, -94.1799) knots 0 0 0 0 1 1 1 1
  spline S981 degree 3 poles (9.9998, -94.1799) (10.0685, -94.1664) (10.0679, -94.1615) (9.9951, -94.1629) knots 0 0 0 0 1 1 1 1
  spline S982 degree 3 poles (9.9951, -94.1629) (9.9224, -94.1643) (9.8912, -94.1757) (9.9134, -94.193) knots 0 0 0 0 1 1 1 1
  spline S983 degree 3 poles (4.1247, -101.8429) (4.1553, -101.8668) (4.1701, -101.8649) (4.1544, -101.8392) knots 0 0 0 0 1 1 1 1
  spline S984 degree 3 poles (4.1544, -101.8392) (4.1415, -101.8157) (4.1143, -101.7989) (4.0994, -101.8007) knots 0 0 0 0 1 1 1 1
  spline S985 degree 3 poles (4.0994, -101.8007) (4.0818, -101.8004) (4.092, -101.8218) (4.1247, -101.8429) knots 0 0 0 0 1 1 1 1
  spline S986 degree 3 poles (13.7889, -89.4447) (13.8235, -89.4404) (13.8493, -89.4247) (13.8474, -89.4098) knots 0 0 0 0 1 1 1 1
  spline S987 degree 3 poles (13.8474, -89.4098) (13.8456, -89.395) (13.8181, -89.3958) (13.788, -89.4171) knots 0 0 0 0 1 1 1 1
  spline S988 degree 3 poles (13.788, -89.4171) (13.7409, -89.443) (13.7415, -89.448) (13.7889, -89.4447) knots 0 0 0 0 1 1 1 1
  spline S989 degree 3 poles (10.1393, -94.1904) (10.1448, -94.1948) (10.1844, -94.1899) (10.2256, -94.1773) knots 0 0 0 0 1 1 1 1
  spline S990 degree 3 poles (10.2256, -94.1773) (10.2943, -94.1638) (10.2937, -94.1589) (10.221, -94.1603) knots 0 0 0 0 1 1 1 1
  spline S991 degree 3 poles (10.221, -94.1603) (10.1483, -94.1617) (10.117, -94.1731) (10.1393, -94.1904) knots 0 0 0 0 1 1 1 1
  spline S992 degree 3 poles (10.9813, -93.1471) (11.0126, -93.1357) (11.0525, -93.1132) (11.0634, -93.0993) knots 0 0 0 0 1 1 1 1
  spline S993 degree 3 poles (11.0634, -93.0993) (11.0764, -93.0826) (11.056, -93.0801) (11.0247, -93.0915) knots 0 0 0 0 1 1 1 1
  spline S994 degree 3 poles (11.0247, -93.0915) (10.9934, -93.1029) (10.9557, -93.1226) (10.9426, -93.1393) knots 0 0 0 0 1 1 1 1
  spline S995 degree 3 poles (10.9426, -93.1393) (10.9318, -93.1532) (10.95, -93.1585) (10.9813, -93.1471) knots 0 0 0 0 1 1 1 1
  spline S996 degree 3 poles (12.7088, -90.9646) (12.7629, -90.9755) (12.7886, -91) (12.7974, -91.0517) knots 0 0 0 0 1 1 1 1
  spline S997 degree 3 poles (12.7974, -91.0517) (12.8103, -91.1155) (12.8158, -91.1198) (12.8549, -91.0698) knots 0 0 0 0 1 1 1 1
  spline S998 degree 3 poles (12.8549, -91.0698) (12.8767, -91.042) (12.8801, -91.0089) (12.8591, -91.0014) knots 0 0 0 0 1 1 1 1
  spline S999 degree 3 poles (12.8591, -91.0014) (12.8409, -90.9961) (12.8212, -90.9583) (12.8212, -90.9181) knots 0 0 0 0 1 1 1 1
  spline S1000 degree 3 poles (12.8212, -90.9181) (12.8189, -90.8581) (12.8133, -90.8537) (12.7984, -90.8958) knots 0 0 0 0 1 1 1 1